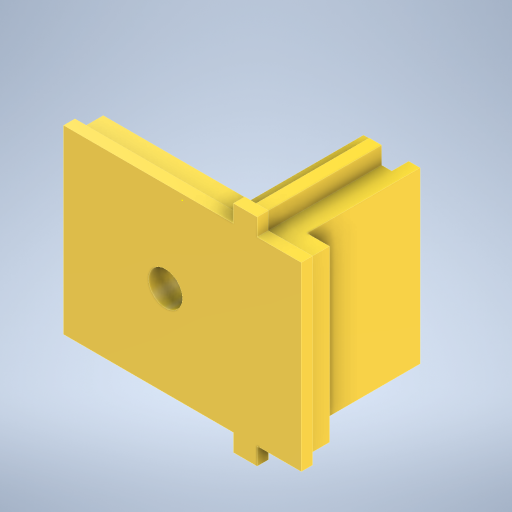
# Autodesk Inventor part: peca2v2
Saved by Autodesk Inventor 2024 (Build 280153000, 153)
## iProperties
Created: 2023-10-22
Part Number: peca2v2
Material: Genérico
Document SubType Name: Modeling
Designer: Daniel
Density: 1 g/cm^3
Appearance: Glossy - Gold
Author: Daniel
Autodesk Inventor part; units mm, degrees
ref_plane "YZ Plane" through (0, 0, 0) normal (1, 0, 0) x (0, 1, 0)
ref_plane "XZ Plane" through (0, 0, 0) normal (0, 1, 0) x (-1, 0, 0)
ref_plane "XY Plane" through (0, 0, 0) normal (0, 0, 1) x (1, 0, 0)
sketch "Esboço1" plane through (0, 0, 0) normal (0, 0, 1) x (1, 0, 0)
  line L0 (-10, 7.5) -> (10, 7.5)
  line L1 (10, 7.5) -> (10, -7.5)
  line L2 (10, -7.5) -> (-10, -7.5)
  line L3 (-10, -7.5) -> (-10, 7.5)
  line L4 (-10, 7.5) -> (10, -7.5) construction
  line L5 (10, 7.5) -> (-10, -7.5) construction
  circle A0 centre (-1.5, 0) radius 1.5
  point P0 (0, 0)
  dimension "d0" = 20
  dimension "d1" = 15
  dimension "d13" = 3
  dimension "d14" = 1.5
  dimension "d15" = 7.5
  constraints: 12 end point, 2 midpoint, 2 parallel, 1 centre point, 1 horizontal, 1 perpendicular
  measures "d0" distance of L0.start L0.end
  measures "d1" distance of L2.end L0.start
  measures "d13" diameter of A0
  measures "d14" distance of point (0, 0) A0.centre
  measures "d15" distance from line of L2 A0.centre
extrude "Extrusão1" add sketch "Esboço1" against normal blind 3
sketch "Esboço2" plane through (0, 0, -3) normal (0, 0, -1) x (-1, 0, 0)
  line L0 (10, 7.5) -> (-10, 7.5) projected
  line L1 (-4, 7.5) -> (-4, -7.5247)
  line L2 (-7, 7.5) -> (-7, -7.5)
  line L3 (-10, -7.5) -> (10, -7.5) projected
  line L4 (-3, 7.5) -> (-3, -7.5247)
  line L5 (-8, 7.5) -> (-8, -7.5)
  point P0 (0, 0)
  point P1 (0, 0)
  point P2 (-3, -7.5)
  point P3 (-4, -7.5)
  dimension "d6" = 3
  dimension "d7" = 1
  dimension "d8" = 1
  dimension "d16" = 7
  constraints: 8 end point, 3 point on line, 2 parallel, 2 vertical
  measures "d6" distance between parallel lines of L2 L1
  measures "d7" distance between parallel lines of L1 L4
  measures "d8" distance between parallel lines of L2 L5
  measures "d16" horizontal distance of L2.start point (0, 0)
extrude "Extrusão2" add sketch "Esboço2" along normal blind 10 contours L4 L3 L1 L0 | L2 L3 L5 L0
sketch "Esboço3" plane through (-10, 7.5, 0) normal (0, 1, 0) x (1, 0, 0)
  point P0 (10, 0)
sketch "Esboço4" plane through (0, 0, -3) normal (0, 0, -1) x (-1, 0, 0)
  line L0 (-7, 7.5) -> (-7, -7.5) projected
  line L1 (-7, -7.5) -> (-4, -7.5) projected
  line L2 (-4, -7.5) -> (-4, 7.5) projected
  line L3 (-4, 7.5) -> (-7, 7.5) projected
  point P0 (0, 0)
extrude "Extrusão3" add sketch "Esboço4" along normal blind 7
sketch "Sketch5" plane through (0, 0, -10) normal (0, 0, -1) x (-1, 0, 0)
  line L0 (-6.1, 0) -> (-6.1, 9.035)
  line L1 (-6.1, 9.035) -> (-5, 9.035)
  line L2 (-5, 9.035) -> (-5, 0)
  line L3 (-3, 7.5) -> (-8, 7.5) projected
  line L4 (-7.6007, 9.235) -> (-6.101, 9.235) projected
  line L5 (-4, 3.5) -> (-4, 7.373) projected
  line L6 (-7, 7.373) -> (-7, 3.5) projected
  line L7 (-6.101, -10.265) -> (-7.6007, -10.265) projected
  line L8 (-11.7517, 0) -> (0.9741, 0)
  line L9 (-6.1, 0) -> (-6.1, -9.035)
  line L10 (-6.1, -9.035) -> (-5, -9.035)
  line L11 (-5, -9.035) -> (-5, 0)
  point P0 (0, 0)
  dimension "d21" = 0.2
  dimension "d22" = 1
  dimension "d23" = 0.9
  constraints: 14 end point, 2 point on line, 2 symmetric about line, 1 horizontal, 1 parallel
  measures "d21" distance between parallel lines of L4 L1
  measures "d22" distance between parallel lines of L5 L2
  measures "d23" distance between parallel lines of L6 L0
extrude "Extrusion4" add sketch "Sketch5" against normal blind 10
sketch "Sketch7" plane through (0, 0, 0) normal (0, 0, 1) x (1, 0, 0)
  circle A0 centre (-1.5, 0) radius 1.5 projected
  line L0 (6.1, -7.5) -> (10, -7.5) projected
  line L1 (10, -7.5) -> (10, 7.5) projected
  line L2 (10, 7.5) -> (6.1, 7.5) projected
  line L3 (6.1, 7.5) -> (6.1, 9.035) projected
  line L4 (6.1, 9.035) -> (5, 9.035) projected
  line L5 (5, 9.035) -> (5, 7.5) projected
  line L6 (5, 7.5) -> (-10, 7.5) projected
  line L7 (-10, 7.5) -> (-10, -7.5) projected
  line L8 (-10, -7.5) -> (5, -7.5) projected
  line L9 (5, -7.5) -> (5, -9.035) projected
  line L10 (5, -9.035) -> (6.1, -9.035) projected
  line L11 (6.1, -9.035) -> (6.1, -7.5) projected
  line L12 (10.5, 8) -> (10.5, -8)
  line L13 (10.5, -8) -> (6.6, -8)
  line L14 (6.6, -8) -> (6.6, -9.535)
  line L15 (6.6, -9.535) -> (4.5, -9.535)
  line L16 (4.5, -9.535) -> (4.5, -8)
  line L17 (4.5, -8) -> (-10.5, -8)
  line L18 (-10.5, -8) -> (-10.5, 8)
  line L19 (-10.5, 8) -> (4.5, 8)
  line L20 (4.5, 8) -> (4.5, 9.535)
  line L21 (4.5, 9.535) -> (6.6, 9.535)
  line L22 (6.6, 9.535) -> (6.6, 8)
  line L23 (6.6, 8) -> (10.5, 8)
  circle A1 centre (-1.5, 0) radius 1.5
  point P0 (0, 0)
  dimension "d32" = 0.5
  constraints: 24 end point, 1 centre point, 1 coincident, 1 concentric, 11 other
  measures "d32" distance between parallel lines of L1 L12
extrude "Extrusion6" add sketch "Sketch7" against normal blind 1 contours L12 L13 L14 L15 L16 L17 L18 L19 L20 L21 L22 L23
sketch "Sketch8" plane through (0, 0, -10) normal (0, 0, -1) x (-1, 0, 0)
  line L0 (-6.1, 7.5) -> (-7, 7.5) projected
  line L1 (-7, -7.5) -> (-7, 7.5) projected
  line L2 (-7, -7.5) -> (-6.1, -7.5) projected
  line L3 (-6.1, -7.5) -> (-6.1, -9.035) projected
  line L4 (-6.1, -9.035) -> (-5, -9.035) projected
  line L5 (-5, -9.035) -> (-5, -7.5) projected
  line L6 (-5, -7.5) -> (-4, -7.5) projected
  line L7 (-4, 7.5) -> (-4, -7.5) projected
  line L8 (-4, 7.5) -> (-5, 7.5) projected
  line L9 (-5, 7.5) -> (-5, 9.035) projected
  line L10 (-5, 9.035) -> (-6.1, 9.035) projected
  line L11 (-6.1, 9.035) -> (-6.1, 7.5) projected
  point P0 (0, 0)
extrude "Extrusion7" add sketch "Sketch8" along normal blind 1.5
